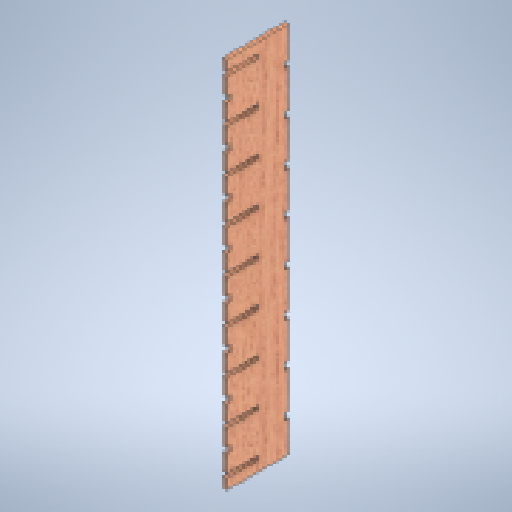
# Autodesk Inventor part: Separators
Saved by Autodesk Inventor 2024 (Build 280153000, 153)
## iProperties
Created: 2023-07-19
Part Number: Separators
Material: Generic
Document SubType Name: Modeling
Designer: Bruno
Density: 1 g/cm^3
Appearance: Default
Author: Bruno
Autodesk Inventor part; units mm, degrees
ref_plane "YZ Plane" through (0, 0, 0) normal (1, 0, 0) x (0, 1, 0)
ref_plane "XZ Plane" through (0, 0, 0) normal (0, 1, 0) x (-1, 0, 0)
ref_plane "XY Plane" through (0, 0, 0) normal (0, 0, 1) x (1, 0, 0)
sketch "Sketch1" plane through (0, 0, 0) normal (1, 0, 0) x (0, 1, 0)
  line L0 (0, 66) -> (0, 0)
  line L1 (15, 63) -> (15, 33)
  line L2 (15, 33) -> (16.55, 33)
  line L3 (16.55, 33) -> (18.1, 33)
  line L4 (18.1, 33) -> (18.1, 63)
  line L5 (18.1, 63) -> (31.55, 63)
  line L6 (31.55, 63) -> (31.55, 60)
  line L7 (31.55, 60) -> (36.55, 60)
  line L8 (36.55, 60) -> (36.55, 63)
  line L9 (36.55, 63) -> (50, 63)
  line L10 (50, 63) -> (50, 33)
  line L11 (50, 33) -> (51.55, 33)
  line L12 (16.55, 3) -> (31.55, 3)
  line L13 (31.55, 3) -> (31.55, 6)
  line L14 (31.55, 6) -> (36.55, 6)
  line L15 (36.55, 6) -> (36.55, 3)
  line L16 (36.55, 3) -> (51.55, 3)
  line L17 (51.55, 33) -> (53.1, 33)
  line L18 (53.1, 33) -> (53.1, 63)
  line L19 (53.1, 63) -> (66.55, 63)
  line L20 (66.55, 60) -> (71.55, 60)
  line L21 (66.55, 63) -> (66.55, 60)
  line L22 (71.55, 60) -> (71.55, 63)
  line L23 (71.55, 63) -> (85, 63)
  line L24 (85, 63) -> (85, 33)
  line L25 (85, 33) -> (86.55, 33)
  line L26 (71.55, 3) -> (86.55, 3)
  line L27 (66.55, 6) -> (71.55, 6)
  line L28 (71.55, 6) -> (71.55, 3)
  line L29 (66.55, 3) -> (66.55, 6)
  line L30 (51.55, 3) -> (66.55, 3)
  line L31 (86.55, 33) -> (88.1, 33)
  line L32 (88.1, 33) -> (88.1, 63)
  line L33 (88.1, 63) -> (101.55, 63)
  line L34 (101.55, 60) -> (106.55, 60)
  line L35 (101.55, 63) -> (101.55, 60)
  line L36 (106.55, 60) -> (106.55, 63)
  line L37 (106.55, 63) -> (120, 63)
  line L38 (120, 63) -> (120, 33)
  line L39 (120, 33) -> (121.55, 33)
  line L40 (106.55, 3) -> (121.55, 3)
  line L41 (101.55, 6) -> (106.55, 6)
  line L42 (106.55, 6) -> (106.55, 3)
  line L43 (101.55, 3) -> (101.55, 6)
  line L44 (86.55, 3) -> (101.55, 3)
  line L45 (121.55, 33) -> (123.1, 33)
  line L46 (123.1, 33) -> (123.1, 63)
  line L47 (123.1, 63) -> (136.55, 63)
  line L48 (136.55, 60) -> (141.55, 60)
  line L49 (136.55, 63) -> (136.55, 60)
  line L50 (141.55, 60) -> (141.55, 63)
  line L51 (141.55, 63) -> (155, 63)
  line L52 (155, 63) -> (155, 33)
  line L53 (155, 33) -> (156.55, 33)
  line L54 (141.55, 3) -> (156.55, 3)
  line L55 (136.55, 6) -> (141.55, 6)
  line L56 (141.55, 6) -> (141.55, 3)
  line L57 (136.55, 3) -> (136.55, 6)
  line L58 (121.55, 3) -> (136.55, 3)
  line L59 (156.55, 33) -> (158.1, 33)
  line L60 (158.1, 33) -> (158.1, 63)
  line L61 (158.1, 63) -> (171.55, 63)
  line L62 (171.55, 60) -> (176.55, 60)
  line L63 (171.55, 63) -> (171.55, 60)
  line L64 (176.55, 60) -> (176.55, 63)
  line L65 (176.55, 63) -> (190, 63)
  line L66 (190, 63) -> (190, 33)
  line L67 (190, 33) -> (191.55, 33)
  line L68 (176.55, 3) -> (191.55, 3)
  line L69 (171.55, 6) -> (176.55, 6)
  line L70 (176.55, 6) -> (176.55, 3)
  line L71 (171.55, 3) -> (171.55, 6)
  line L72 (156.55, 3) -> (171.55, 3)
  line L73 (191.55, 33) -> (193.1, 33)
  line L74 (193.1, 33) -> (193.1, 63)
  line L75 (193.1, 63) -> (206.55, 63)
  line L76 (206.55, 60) -> (211.55, 60)
  line L77 (206.55, 63) -> (206.55, 60)
  line L78 (211.55, 60) -> (211.55, 63)
  line L79 (211.55, 63) -> (225, 63)
  line L80 (225, 63) -> (225, 33)
  line L81 (225, 33) -> (226.55, 33)
  line L82 (211.55, 3) -> (226.55, 3)
  line L83 (206.55, 6) -> (211.55, 6)
  line L84 (211.55, 6) -> (211.55, 3)
  line L85 (206.55, 3) -> (206.55, 6)
  line L86 (191.55, 3) -> (206.55, 3)
  line L87 (226.55, 33) -> (228.1, 33)
  line L88 (228.1, 33) -> (228.1, 63)
  line L89 (228.1, 63) -> (241.55, 63)
  line L90 (241.55, 60) -> (246.55, 60)
  line L91 (241.55, 63) -> (241.55, 60)
  line L92 (246.55, 60) -> (246.55, 63)
  line L93 (246.55, 63) -> (260, 63)
  line L94 (260, 63) -> (260, 33)
  line L95 (260, 33) -> (261.55, 33)
  line L96 (246.55, 3) -> (261.55, 3)
  line L97 (241.55, 6) -> (246.55, 6)
  line L98 (246.55, 6) -> (246.55, 3)
  line L99 (241.55, 3) -> (241.55, 6)
  line L100 (226.55, 3) -> (241.55, 3)
  line L101 (261.55, 33) -> (263.1, 33)
  line L102 (263.1, 33) -> (263.1, 63)
  line L103 (263.1, 63) -> (276.55, 63)
  line L104 (276.55, 60) -> (281.55, 60)
  line L105 (276.55, 63) -> (276.55, 60)
  line L106 (281.55, 60) -> (281.55, 63)
  line L107 (281.55, 63) -> (295, 63)
  line L108 (295, 63) -> (295, 33)
  line L109 (295, 33) -> (296.55, 33)
  line L110 (281.55, 3) -> (296.55, 3)
  line L111 (276.55, 6) -> (281.55, 6)
  line L112 (281.55, 6) -> (281.55, 3)
  line L113 (276.55, 3) -> (276.55, 6)
  line L114 (261.55, 3) -> (276.55, 3)
  line L115 (156.55, 3) -> (156.55, 33) construction
  line L116 (15, 3) -> (16.55, 3)
  line L117 (0, 66) -> (8, 66)
  line L118 (8, 66) -> (8, 63)
  line L119 (8, 63) -> (15, 63)
  line L120 (0, 0) -> (8, 0)
  line L121 (8, 0) -> (8, 3)
  line L122 (8, 3) -> (16.55, 3)
  line L123 (313.1, 66) -> (313.1, 0)
  line L124 (298.1, 63) -> (298.1, 33)
  line L125 (298.1, 33) -> (296.55, 33)
  line L126 (298.1, 3) -> (296.55, 3)
  line L127 (313.1, 66) -> (305.1, 66)
  line L128 (305.1, 66) -> (305.1, 63)
  line L129 (305.1, 63) -> (298.1, 63)
  line L130 (313.1, 0) -> (305.1, 0)
  line L131 (305.1, 0) -> (305.1, 3)
  line L132 (305.1, 3) -> (296.55, 3)
  line L133 (298.1, 21) -> (302.1, 21)
  line L134 (302.1, 21) -> (302.1, 11)
  line L135 (302.1, 11) -> (298.1, 11)
  line L136 (298.1, 11) -> (298.1, 21)
  point P0 (15.775, 33)
  point P1 (297.325, 33)
  dimension "d36" = 1.55
  dimension "d37" = 1.55
  dimension "d39" = 5
  dimension "d41" = 1.55
  dimension "d42" = 35
  dimension "d43" = 5
  dimension "d45" = 3
  dimension "d46" = 35
  dimension "d51" = 35
  dimension "d61" = 30
  dimension "d62" = 60
  dimension "d63" = 3
  dimension "d66" = 3
  dimension "d67" = 8
  dimension "d68" = 7
  dimension "d69" = 4
  dimension "d70" = 10
  dimension "d71" = 8
  constraints: 274 end point, 48 point on line, 14 perpendicular, 11 symmetric about line, 7 horizontal, 5 collinear, 4 vertical alignment, 3 parallel, 2 coincident, 2 vertical, 1 horizontal alignment, 1 midpoint, 209 other
  measures "d36" distance of L1.end L2.end
  measures "d37" distance of L2.end L3.end
  measures "d39" distance of L6.end L7.end
  measures "d41" distance of L10.end L11.end
  measures "d42" distance of L11.end L2.end
  measures "d43" distance of L13.end L14.end
  measures "d45" distance of L12.end L13.end
  measures "d46" distance of L12.start L16.end
  measures "d51" distance of L3.end L17.end
  measures "d61" distance from line of L5 point (15.775, 33)
  measures "d62" distance between parallel lines of L12 L5
  measures "d63" distance of L7.end L8.end
  measures "d66" distance between parallel lines of L117 L5
  measures "d67" distance of L0.start L117.end
  measures "d68" distance of L118.end L1.start
  measures "d69" distance of L134.end L135.end
  measures "d70" distance of L133.end L134.end
  measures "d71" distance between parallel lines of L132 L135
extrude "Extrusion1" add sketch "Sketch1" along normal blind 3
body "Solid1"
